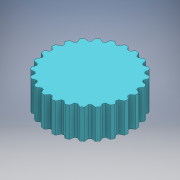
# Autodesk Inventor part: 02CybertruckWheels
Saved by Autodesk Inventor 2018 (Build 220112000, 112)
## iProperties
Created: 2020-06-23
Part Number: 02CybertruckWheels
Material: Generic
Document SubType Name: Modeling
Designer: Ivan
Density: 1 g/cm^3
Appearance: Default
Author: Ivan
Autodesk Inventor part; units mm, degrees
ref_plane "YZ Plane" through (0, 0, 0) normal (1, 0, 0) x (0, 1, 0)
ref_plane "XZ Plane" through (0, 0, 0) normal (0, 1, 0) x (-1, 0, 0)
ref_plane "XY Plane" through (0, 0, 0) normal (0, 0, 1) x (1, 0, 0)
sketch "Sketch1" plane through (0, 0, 0) normal (0, 0, 1) x (1, 0, 0)
  circle A0 centre (0, 0) radius 425
  dimension "d0" = 850
  constraints: 1 centre point, 1 coincident
  measures "d0" diameter of A0
extrude "Extrusion1" add sketch "Sketch1" along normal blind 300
sketch "Sketch2" plane through (0, 0, 300) normal (0, 0, 1) x (1, 0, 0)
  circle A0 centre (0, 0) radius 425 projected
  line L0 (0, 425) -> (40, 425)
  line L1 (40, 425) -> (11.0746, 390.528)
  line L2 (0, 425) -> (0, 390.528) construction
  line L3 (11.0746, 390.528) -> (0, 390.528)
  line L4 (0, 425) -> (-40, 425)
  line L5 (-40, 425) -> (-11.0746, 390.528)
  line L6 (-11.0746, 390.528) -> (0, 390.528)
  line L7 (109.9981, 410.5185) -> (71.3611, 420.8712)
  line L8 (71.3611, 420.8712) -> (90.3789, 380.0874)
  line L9 (90.3789, 380.0874) -> (101.0761, 377.2211)
  line L10 (111.7733, 374.3548) -> (101.0761, 377.2211)
  line L11 (148.6351, 400.1657) -> (111.7733, 374.3548)
  line L12 (109.9981, 410.5185) -> (148.6351, 400.1657)
  line L13 (212.5, 368.0608) -> (177.859, 388.0608)
  line L14 (177.859, 388.0608) -> (185.6732, 343.7444)
  line L15 (185.6732, 343.7444) -> (195.264, 338.2072)
  line L16 (204.8548, 332.6699) -> (195.264, 338.2072)
  line L17 (247.141, 348.0608) -> (204.8548, 332.6699)
  line L18 (212.5, 368.0608) -> (247.141, 348.0608)
  line L19 (300.5204, 300.5204) -> (272.2361, 328.8047)
  line L20 (272.2361, 328.8047) -> (268.3141, 283.9759)
  line L21 (268.3141, 283.9759) -> (276.145, 276.145)
  line L22 (283.9759, 268.3141) -> (276.145, 276.145)
  line L23 (328.8047, 272.2361) -> (283.9759, 268.3141)
  line L24 (300.5204, 300.5204) -> (328.8047, 272.2361)
  line L25 (368.0608, 212.5) -> (348.0608, 247.141)
  line L26 (348.0608, 247.141) -> (332.6699, 204.8548)
  line L27 (332.6699, 204.8548) -> (338.2072, 195.264)
  line L28 (343.7444, 185.6732) -> (338.2072, 195.264)
  line L29 (388.0608, 177.859) -> (343.7444, 185.6732)
  line L30 (368.0608, 212.5) -> (388.0608, 177.859)
  line L31 (410.5185, 109.9981) -> (400.1657, 148.6351)
  line L32 (400.1657, 148.6351) -> (374.3548, 111.7733)
  line L33 (374.3548, 111.7733) -> (377.2211, 101.0761)
  line L34 (380.0874, 90.3789) -> (377.2211, 101.0761)
  line L35 (420.8712, 71.3611) -> (380.0874, 90.3789)
  line L36 (410.5185, 109.9981) -> (420.8712, 71.3611)
  line L37 (425, 0) -> (425, 40)
  line L38 (425, 40) -> (390.528, 11.0746)
  line L39 (390.528, 11.0746) -> (390.528, 0)
  line L40 (390.528, -11.0746) -> (390.528, 0)
  line L41 (425, -40) -> (390.528, -11.0746)
  line L42 (425, 0) -> (425, -40)
  line L43 (410.5185, -109.9981) -> (420.8712, -71.3611)
  line L44 (420.8712, -71.3611) -> (380.0874, -90.3789)
  line L45 (380.0874, -90.3789) -> (377.2211, -101.0761)
  line L46 (374.3548, -111.7733) -> (377.2211, -101.0761)
  line L47 (400.1657, -148.6351) -> (374.3548, -111.7733)
  line L48 (410.5185, -109.9981) -> (400.1657, -148.6351)
  line L49 (368.0608, -212.5) -> (388.0608, -177.859)
  line L50 (388.0608, -177.859) -> (343.7444, -185.6732)
  line L51 (343.7444, -185.6732) -> (338.2072, -195.264)
  line L52 (332.6699, -204.8548) -> (338.2072, -195.264)
  line L53 (348.0608, -247.141) -> (332.6699, -204.8548)
  line L54 (368.0608, -212.5) -> (348.0608, -247.141)
  line L55 (300.5204, -300.5204) -> (328.8047, -272.2361)
  line L56 (328.8047, -272.2361) -> (283.9759, -268.3141)
  line L57 (283.9759, -268.3141) -> (276.145, -276.145)
  line L58 (268.3141, -283.9759) -> (276.145, -276.145)
  line L59 (272.2361, -328.8047) -> (268.3141, -283.9759)
  line L60 (300.5204, -300.5204) -> (272.2361, -328.8047)
  line L61 (212.5, -368.0608) -> (247.141, -348.0608)
  line L62 (247.141, -348.0608) -> (204.8548, -332.6699)
  line L63 (204.8548, -332.6699) -> (195.264, -338.2072)
  line L64 (185.6732, -343.7444) -> (195.264, -338.2072)
  line L65 (177.859, -388.0608) -> (185.6732, -343.7444)
  line L66 (212.5, -368.0608) -> (177.859, -388.0608)
  line L67 (109.9981, -410.5185) -> (148.6351, -400.1657)
  line L68 (148.6351, -400.1657) -> (111.7733, -374.3548)
  line L69 (111.7733, -374.3548) -> (101.0761, -377.2211)
  line L70 (90.3789, -380.0874) -> (101.0761, -377.2211)
  line L71 (71.3611, -420.8712) -> (90.3789, -380.0874)
  line L72 (109.9981, -410.5185) -> (71.3611, -420.8712)
  line L73 (0, -425) -> (40, -425)
  line L74 (40, -425) -> (11.0746, -390.528)
  line L75 (11.0746, -390.528) -> (0, -390.528)
  line L76 (-11.0746, -390.528) -> (0, -390.528)
  line L77 (-40, -425) -> (-11.0746, -390.528)
  line L78 (0, -425) -> (-40, -425)
  line L79 (-109.9981, -410.5185) -> (-71.3611, -420.8712)
  line L80 (-71.3611, -420.8712) -> (-90.3789, -380.0874)
  line L81 (-90.3789, -380.0874) -> (-101.0761, -377.2211)
  line L82 (-111.7733, -374.3548) -> (-101.0761, -377.2211)
  line L83 (-148.6351, -400.1657) -> (-111.7733, -374.3548)
  line L84 (-109.9981, -410.5185) -> (-148.6351, -400.1657)
  line L85 (-212.5, -368.0608) -> (-177.859, -388.0608)
  line L86 (-177.859, -388.0608) -> (-185.6732, -343.7444)
  line L87 (-185.6732, -343.7444) -> (-195.264, -338.2072)
  line L88 (-204.8548, -332.6699) -> (-195.264, -338.2072)
  line L89 (-247.141, -348.0608) -> (-204.8548, -332.6699)
  line L90 (-212.5, -368.0608) -> (-247.141, -348.0608)
  line L91 (-300.5204, -300.5204) -> (-272.2361, -328.8047)
  line L92 (-272.2361, -328.8047) -> (-268.3141, -283.9759)
  line L93 (-268.3141, -283.9759) -> (-276.145, -276.145)
  line L94 (-283.9759, -268.3141) -> (-276.145, -276.145)
  line L95 (-328.8047, -272.2361) -> (-283.9759, -268.3141)
  line L96 (-300.5204, -300.5204) -> (-328.8047, -272.2361)
  line L97 (-368.0608, -212.5) -> (-348.0608, -247.141)
  line L98 (-348.0608, -247.141) -> (-332.6699, -204.8548)
  line L99 (-332.6699, -204.8548) -> (-338.2072, -195.264)
  line L100 (-343.7444, -185.6732) -> (-338.2072, -195.264)
  line L101 (-388.0608, -177.859) -> (-343.7444, -185.6732)
  line L102 (-368.0608, -212.5) -> (-388.0608, -177.859)
  line L103 (-410.5185, -109.9981) -> (-400.1657, -148.6351)
  line L104 (-400.1657, -148.6351) -> (-374.3548, -111.7733)
  line L105 (-374.3548, -111.7733) -> (-377.2211, -101.0761)
  line L106 (-380.0874, -90.3789) -> (-377.2211, -101.0761)
  line L107 (-420.8712, -71.3611) -> (-380.0874, -90.3789)
  line L108 (-410.5185, -109.9981) -> (-420.8712, -71.3611)
  line L109 (-425, 0) -> (-425, -40)
  line L110 (-425, -40) -> (-390.528, -11.0746)
  line L111 (-390.528, -11.0746) -> (-390.528, 0)
  line L112 (-390.528, 11.0746) -> (-390.528, 0)
  line L113 (-425, 40) -> (-390.528, 11.0746)
  line L114 (-425, 0) -> (-425, 40)
  line L115 (-410.5185, 109.9981) -> (-420.8712, 71.3611)
  line L116 (-420.8712, 71.3611) -> (-380.0874, 90.3789)
  line L117 (-380.0874, 90.3789) -> (-377.2211, 101.0761)
  line L118 (-374.3548, 111.7733) -> (-377.2211, 101.0761)
  line L119 (-400.1657, 148.6351) -> (-374.3548, 111.7733)
  line L120 (-410.5185, 109.9981) -> (-400.1657, 148.6351)
  line L121 (-368.0608, 212.5) -> (-388.0608, 177.859)
  line L122 (-388.0608, 177.859) -> (-343.7444, 185.6732)
  line L123 (-343.7444, 185.6732) -> (-338.2072, 195.264)
  line L124 (-332.6699, 204.8548) -> (-338.2072, 195.264)
  line L125 (-348.0608, 247.141) -> (-332.6699, 204.8548)
  line L126 (-368.0608, 212.5) -> (-348.0608, 247.141)
  line L127 (-300.5204, 300.5204) -> (-328.8047, 272.2361)
  line L128 (-328.8047, 272.2361) -> (-283.9759, 268.3141)
  line L129 (-283.9759, 268.3141) -> (-276.145, 276.145)
  line L130 (-268.3141, 283.9759) -> (-276.145, 276.145)
  line L131 (-272.2361, 328.8047) -> (-268.3141, 283.9759)
  line L132 (-300.5204, 300.5204) -> (-272.2361, 328.8047)
  line L133 (-212.5, 368.0608) -> (-247.141, 348.0608)
  line L134 (-247.141, 348.0608) -> (-204.8548, 332.6699)
  line L135 (-204.8548, 332.6699) -> (-195.264, 338.2072)
  line L136 (-185.6732, 343.7444) -> (-195.264, 338.2072)
  line L137 (-177.859, 388.0608) -> (-185.6732, 343.7444)
  line L138 (-212.5, 368.0608) -> (-177.859, 388.0608)
  line L139 (-109.9981, 410.5185) -> (-148.6351, 400.1657)
  line L140 (-148.6351, 400.1657) -> (-111.7733, 374.3548)
  line L141 (-111.7733, 374.3548) -> (-101.0761, 377.2211)
  line L142 (-90.3789, 380.0874) -> (-101.0761, 377.2211)
  line L143 (-71.3611, 420.8712) -> (-90.3789, 380.0874)
  line L144 (-109.9981, 410.5185) -> (-71.3611, 420.8712)
  dimension "d3" = 40
  dimension "d4" = 45
  dimension "d5" = 50
  dimension "d8" = 360
  constraints: 290 end point, 2 coincident, 2 horizontal, 2 symmetric about line, 1 perpendicular, 1 vertical, 1 vertical alignment, 311 other
  measures "d3" distance of L0.start L0.end
  measures "d4" distance of L0.end L1.end
  measures "d5" angle of L0 L1
extrude "Extrusion2" cut sketch "Sketch2" against normal up to surface (300 mm away) contours A0 L41 L40 L39 L38 | L42 L41 A0 | A0 L38 L37 | L35 L34 L33 L32 A0 | A0 L36 L35 | L44 L43 A0 | A0 L47 L46 L45 L44 | A0 L32 L31 | L48 L47 A0 | L29 L28 L27 L26 A0 | A0 L30 L29 | L50 L49 A0 | A0 L53 L52 L51 L50 | A0 L26 L25 | L54 L53 A0 | L23 L22 L21 L20 A0 | A0 L24 L23 | L56 L55 A0 | A0 L59 L58 L57 L56 | A0 L20 L19 | L60 L59 A0 | L17 L16 L15 L14 A0 | A0 L18 L17 | L62 L61 A0 | A0 L65 L64 L63 L62 | A0 L14 L13 | L66 L65 A0 | L11 L10 L9 L8 A0 | A0 L12 L11 | L68 L67 A0 | A0 L71 L70 L69 L68 | A0 L8 L7 | L72 L71 A0 | L1 L3 L6 L5 A0 | A0 L0 L1 | L74 L73 A0 | A0 L77 L76 L75 L74 | A0 L5 L4 | L78 L77 A0 | L143 L142 L141 L140 A0 | A0 L144 L143 | L80 L79 A0 | A0 L83 L82 L81 L80 | A0 L140 L139 | L84 L83 A0 | L137 L136 L135 L134 A0 | A0 L138 L137 | L86 L85 A0 | A0 L89 L88 L87 L86 | A0 L134 L133 | L90 L89 A0 | L131 L130 L129 L128 A0 | A0 L132 L131 | L92 L91 A0 | A0 L95 L94 L93 L92 | A0 L128 L127 | L96 L95 A0 | L125 L124 L123 L122 A0 | A0 L126 L125 | L98 L97 A0 | A0 L101 L100 L99 L98 | A0 L122 L121 | L102 L101 A0 | L119 L118 L117 L116 A0 | A0 L120 L119 | L104 L103 A0 | A0 L107 L106 L105 L104 | A0 L116 L115 | L108 L107 A0 | L113 L112 L111 L110 A0 | A0 L114 L113 | L110 L109 A0
body "Solid1"
